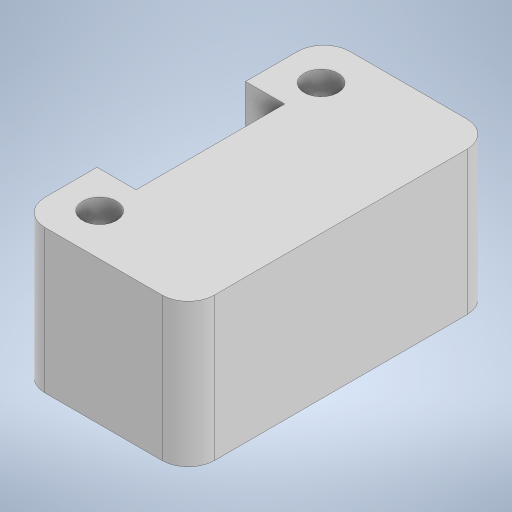
# Autodesk Inventor part: стойки для драйверов
Saved by Autodesk Inventor 2023 (Build 270158000, 158)
## iProperties
Created: 2026-02-07
Part Number: стойки для драйверов
Material: Типовые
Document SubType Name: Modeling
Designer: garin
Density: 1 g/cm^3
Appearance: По умолчанию
Author: garin
Autodesk Inventor part; units mm, degrees
ref_plane "YZ Plane" through (0, 0, 0) normal (1, 0, 0) x (0, 1, 0)
ref_plane "XZ Plane" through (0, 0, 0) normal (0, 1, 0) x (-1, 0, 0)
ref_plane "XY Plane" through (0, 0, 0) normal (0, 0, 1) x (1, 0, 0)
sketch "Эскиз1" plane through (0, 0, 0) normal (0, 1, 0) x (-1, 0, 0)
  circle A0 centre (0, 8.5) radius 1.3
  circle A1 centre (0, -8.5) radius 1.3
  line L0 (0, 5.7) -> (3, 5.7)
  line L1 (3, 5.7) -> (3, 11.7)
  line L2 (3, 11.7) -> (-10, 11.7)
  line L3 (-10, 11.7) -> (-10, 0)
  line L4 (5.8356, 0) -> (-16.6075, 0) construction
  line L5 (0, 5.7) -> (0, 0)
  circle A2 centre (0, -8.5) radius 1.3
  line L6 (0, -5.7) -> (3, -5.7)
  line L7 (3, -5.7) -> (3, -11.7)
  line L8 (3, -11.7) -> (-10, -11.7)
  line L9 (-10, -11.7) -> (-10, 0)
  line L10 (0, -5.7) -> (0, 0)
  dimension "d1" = 2.6
  dimension "d2" = 2.6
  dimension "d5" = 3
  dimension "d6" = 6
  dimension "d7" = 13
  constraints: 22 end point, 5 perpendicular, 5 symmetric about line, 3 centre point, 2 coincident, 1 horizontal, 1 other
  measures "d1" diameter of A0
  measures "d2" diameter of A1
  measures "d5" distance of L0.start L0.end
  measures "d6" distance of L0.end L1.end
  measures "d7" distance of L1.end L2.end
extrude "Выдавливание1" add sketch "Эскиз1" along normal blind 11
fillet "Сопряжение1" radius 2 4 edges at (10, 5.5, 11.7) (-3, 5.5, 11.7) (10, 5.5, -11.7) (-3, 5.5, -11.7)
